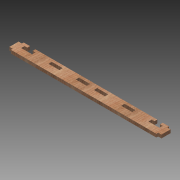
# Autodesk Inventor part: Viga trasera
Saved by Autodesk Inventor 2015 (Build 190159000, 159)
## iProperties
Created: 2016-02-08
Part Number: Viga trasera
Material: Wood (Birch)
Document SubType Name: Modeling
Designer: iberopuebla
Density: 0.55 g/cm^3
Appearance: Birch - Natural Polished
Author: iberopuebla
Autodesk Inventor part; units mm, degrees
ref_plane "YZ Plane" through (0, 0, 0) normal (1, 0, 0) x (0, 1, 0)
ref_plane "XZ Plane" through (0, 0, 0) normal (0, 1, 0) x (-1, 0, 0)
ref_plane "XY Plane" through (0, 0, 0) normal (0, 0, 1) x (1, 0, 0)
sketch "Sketch1" plane through (0, 0, 0) normal (0, 0, 1) x (1, 0, 0)
  line L0 (-2761.2962, 915.5779) -> (-1961.2962, 915.5779)
  line L1 (-1961.2962, 845.5779) -> (-2761.2962, 845.5779)
  line L2 (-2761.2962, 905.5779) -> (-2779.2962, 905.5779)
  line L3 (-2779.2962, 905.5779) -> (-2779.2962, 855.5779)
  line L4 (-2779.2962, 855.5779) -> (-2761.2962, 855.5779)
  line L5 (-1961.2962, 905.5779) -> (-1943.2962, 905.5779)
  line L6 (-1943.2962, 905.5779) -> (-1943.2962, 855.5779)
  line L7 (-1943.2962, 855.5779) -> (-1961.2962, 855.5779)
  line L8 (-1961.2962, 915.5779) -> (-1961.2962, 905.5779)
  line L9 (-1961.2962, 855.5779) -> (-1961.2962, 845.5779)
  line L10 (-2761.2962, 845.5779) -> (-2761.2962, 855.5779)
  line L11 (-2761.2962, 905.5779) -> (-2761.2962, 915.5779)
  point P0 (0, 0)
  dimension "d8" = 800
  dimension "d9" = 70
  dimension "d11" = 50
  dimension "d12" = 18
  dimension "d13" = 18
  dimension "d14" = 50
  dimension "d15" = 10
  dimension "d18" = 800
  dimension "d19" = 10
  dimension "d20" = 10
  constraints: 24 end point, 7 parallel, 4 perpendicular, 3 horizontal
  measures "d8" distance of L0.start L0.end
  measures "d9" distance between parallel lines of L1 L0
  measures "d11" distance of L2.start L4.end
  measures "d12" distance of L3.end L4.end
  measures "d13" distance of L5.start L5.end
  measures "d14" distance of L5.end L6.end
  measures "d15" distance between parallel lines of L0 L5
  measures "d18" distance of L1.start L1.end
  measures "d19" distance between parallel lines of L0 L2
  measures "d20" distance between parallel lines of L1 L4
extrude "Extrusion1" add sketch "Sketch1" along normal blind 18
sketch "Sketch2" plane through (0, 0, 18) normal (0, 0, 1) x (1, 0, 0)
  line L0 (-1961.2962, 905.5779) -> (-1960.1648, 906.7093)
  line L1 (-1961.2962, 905.5779) -> (-1959.6962, 905.5779) construction
  line L2 (-1961.2962, 855.5779) -> (-1960.1648, 854.4466)
  line L3 (-2761.2962, 855.5779) -> (-2762.4276, 854.4466)
  line L4 (-2761.2962, 905.5779) -> (-2762.4276, 906.7093)
  circle A0 centre (-2762.4276, 906.7093) radius 1.6
  circle A1 centre (-2762.4276, 854.4466) radius 1.6
  circle A2 centre (-1960.1648, 906.7093) radius 1.6
  circle A3 centre (-1960.1648, 854.4466) radius 1.6
  line L5 (-1943.2962, 855.5779) -> (-1943.2962, 905.5779) projected
  line L6 (-2779.2962, 905.5779) -> (-2779.2962, 855.5779) projected
  point P0 (0, 0)
  dimension "d21" = 1.6
  dimension "d22" = 45
  dimension "d23" = 3.2
  dimension "d24" = 3.2
  dimension "d25" = 3.2
  dimension "d26" = 3.2
  dimension "d29" = 836
  constraints: 10 end point, 4 centre point, 3 coincident, 3 perpendicular, 1 equal length, 1 horizontal, 1 point on line
  measures "d21" distance of L0.start L0.end
  measures "d22" angle of L1 L0
  measures "d23" diameter of A0
  measures "d24" diameter of A1
  measures "d25" diameter of A2
  measures "d26" diameter of A3
  measures "d29" distance between parallel lines of L5 L6
extrude "Extrusion2" cut sketch "Sketch2" against normal blind 20
sketch "Sketch3" plane through (0, 0, 18) normal (0, 0, 1) x (1, 0, 0)
  line L0 (-2761.2962, 900.5779) -> (-1961.2962, 900.5779)
  line L1 (-1961.2962, 900.5779) -> (-1961.2962, 882.5779)
  line L2 (-1961.2962, 882.5779) -> (-2761.2962, 882.5779)
  line L3 (-2761.2962, 882.5779) -> (-2761.2962, 900.5779)
  line L4 (-2661.2962, 900.5779) -> (-2661.2962, 882.5779)
  line L5 (-2741.2962, 900.5779) -> (-2741.2962, 882.5779)
  line L6 (-2681.2962, 900.5779) -> (-2681.2962, 882.5779)
  line L7 (-2041.2962, 900.5779) -> (-2041.2962, 882.5779)
  line L8 (-1981.2962, 900.5779) -> (-1981.2962, 882.5779)
  line L9 (-2061.2962, 900.5779) -> (-2061.2962, 882.5779)
  line L10 (-2611.2962, 882.5779) -> (-2611.2962, 900.5779)
  line L11 (-2591.2962, 900.5779) -> (-2591.2962, 882.5779)
  line L12 (-2531.2962, 900.5779) -> (-2531.2962, 882.5779)
  line L13 (-2111.2962, 900.5779) -> (-2111.2962, 882.5779)
  line L14 (-2511.2962, 900.5779) -> (-2511.2962, 882.5779)
  line L15 (-2461.2962, 900.5779) -> (-2461.2962, 882.5779)
  line L16 (-2211.2962, 900.5779) -> (-2211.2962, 882.5779)
  line L17 (-2191.2962, 900.5779) -> (-2191.2962, 882.5779)
  line L18 (-2131.2962, 900.5779) -> (-2131.2962, 882.5779)
  line L19 (-2261.2962, 900.5779) -> (-2261.2962, 882.5779)
  line L20 (-2361.2962, 900.5779) -> (-2361.2962, 882.5779)
  line L21 (-2441.2962, 900.5779) -> (-2441.2962, 882.5779)
  line L22 (-2381.2962, 900.5779) -> (-2381.2962, 882.5779)
  line L23 (-2341.2962, 900.5779) -> (-2341.2962, 882.5779)
  line L24 (-2281.2962, 900.5779) -> (-2281.2962, 882.5779)
  line L25 (-1961.2962, 915.5779) -> (-2761.2962, 915.5779) projected
  line L26 (-2761.2962, 915.5779) -> (-2761.2962, 907.8407) projected
  point P0 (0, 0)
  dimension "d54" = 800
  dimension "d55" = 18
  dimension "d56" = 100
  dimension "d57" = 20
  dimension "d58" = 60
  dimension "d59" = 100
  dimension "d60" = 60
  dimension "d61" = 20
  dimension "d62" = 600
  dimension "d63" = 50
  dimension "d64" = 50
  dimension "d65" = 100
  dimension "d66" = 60
  dimension "d67" = 20
  dimension "d68" = 50
  dimension "d69" = 100
  dimension "d70" = 60
  dimension "d71" = 20
  dimension "d72" = 50
  dimension "d73" = 100
  dimension "d74" = 60
  dimension "d75" = 20
  dimension "d76" = 60
  dimension "d77" = 20
  dimension "d78" = 15
  dimension "d79" = 0
  constraints: 46 end point, 22 vertical, 1 parallel, 48 other
  measures "d54" distance of L1.end L3.start
  measures "d55" distance of L1.start L1.end
  measures "d56" distance between parallel lines of L3 L4
  measures "d57" distance between parallel lines of L3 L5
  measures "d58" distance between parallel lines of L6 L5
  measures "d59" distance between parallel lines of L9 L1
  measures "d60" distance between parallel lines of L8 L7
  measures "d61" distance between parallel lines of L9 L7
  measures "d62" distance between parallel lines of L9 L4
  measures "d63" distance between parallel lines of L10 L4
  measures "d64" distance between parallel lines of L13 L9
  measures "d65" distance between parallel lines of L10 L14
  measures "d66" distance from line of L12 L11.start
  measures "d67" distance between parallel lines of L10 L11
  measures "d68" distance between parallel lines of L14 L15
  measures "d69" distance between parallel lines of L13 L16
  measures "d70" distance between parallel lines of L18 L17
  measures "d71" distance between parallel lines of L16 L17
  measures "d72" distance between parallel lines of L16 L19
  measures "d73" distance between parallel lines of L15 L20
  measures "d74" distance between parallel lines of L21 L22
  measures "d75" distance between parallel lines of L15 L21
  measures "d76" distance between parallel lines of L24 L23
  measures "d77" distance between parallel lines of L23 L20
  measures "d79" distance between parallel lines of L3 L26
extrude "Extrusion3" cut sketch "Sketch3" against normal blind 20 contours L0 L6 L2 L5 | L0 L12 L2 L11 | L0 L22 L2 L21 | L0 L24 L2 L23 | L0 L18 L2 L17 | L0 L8 L2 L7
sketch "Sketch4" plane through (0, 0, 18) normal (0, 0, 1) x (1, 0, 0)
  line L0 (-2741.2962, 900.5779) -> (-2740.1648, 899.4466)
  line L1 (-2741.2962, 900.5779) -> (-2739.6962, 900.5779) construction
  line L2 (-2741.2962, 882.5779) -> (-2740.1648, 883.7093)
  line L3 (-2681.2962, 882.5779) -> (-2682.4276, 883.7093)
  line L4 (-2681.2962, 900.5779) -> (-2682.4276, 899.4466)
  line L5 (-2591.2962, 900.5779) -> (-2590.1648, 899.4466)
  line L6 (-2591.2962, 882.5779) -> (-2590.1648, 883.7093)
  line L7 (-2531.2962, 900.5779) -> (-2532.4276, 899.4466)
  line L8 (-2531.2962, 882.5779) -> (-2532.4276, 883.7093)
  line L9 (-2441.2962, 882.5779) -> (-2440.1648, 883.7093)
  line L10 (-2441.2962, 882.5779) -> (-2439.6962, 882.5779) construction
  line L11 (-2441.2962, 900.5779) -> (-2440.1648, 899.4466)
  line L12 (-2381.2962, 900.5779) -> (-2382.4276, 899.4466)
  line L13 (-2381.2962, 882.5779) -> (-2382.4276, 883.7093)
  line L14 (-2341.2962, 900.5779) -> (-2340.1648, 899.4466)
  line L15 (-2341.2962, 882.5779) -> (-2340.1648, 883.7093)
  line L16 (-2281.2962, 900.5779) -> (-2282.4276, 899.4466)
  line L17 (-2281.2962, 882.5779) -> (-2282.4276, 883.7093)
  line L18 (-2191.2962, 900.5779) -> (-2190.1648, 899.4466)
  line L19 (-2191.2962, 882.5779) -> (-2190.1648, 883.7093)
  line L20 (-2131.2962, 900.5779) -> (-2132.4276, 899.4466)
  line L21 (-2131.2962, 882.5779) -> (-2132.4276, 883.7093)
  line L22 (-2041.2962, 900.5779) -> (-2040.1648, 899.4466)
  line L23 (-2041.2962, 882.5779) -> (-2040.1648, 883.7093)
  line L24 (-1981.2962, 900.5779) -> (-1982.4276, 899.4466)
  line L25 (-1981.2962, 882.5779) -> (-1982.4276, 883.7093)
  circle A0 centre (-2040.1648, 899.4466) radius 1.6
  circle A1 centre (-2040.1648, 883.7093) radius 1.6
  circle A2 centre (-1982.4276, 899.4466) radius 1.6
  circle A3 centre (-1982.4276, 883.7093) radius 1.6
  circle A4 centre (-2132.4276, 899.4466) radius 1.6
  circle A5 centre (-2132.4276, 883.7093) radius 1.6
  circle A6 centre (-2190.1648, 899.4466) radius 1.6
  circle A7 centre (-2190.1648, 883.7093) radius 1.6
  circle A8 centre (-2282.4276, 899.4466) radius 1.6
  circle A9 centre (-2282.4276, 883.7093) radius 1.6
  circle A10 centre (-2340.1648, 899.4466) radius 1.6
  circle A11 centre (-2340.1648, 883.7093) radius 1.6
  circle A12 centre (-2382.4276, 899.4466) radius 1.6
  circle A13 centre (-2382.4276, 883.7093) radius 1.6
  circle A14 centre (-2440.1648, 899.4466) radius 1.6
  circle A15 centre (-2440.1648, 883.7093) radius 1.6
  circle A16 centre (-2532.4276, 899.4466) radius 1.6
  circle A17 centre (-2532.4276, 883.7093) radius 1.6
  circle A18 centre (-2590.1648, 899.4466) radius 1.6
  circle A19 centre (-2590.1648, 883.7093) radius 1.6
  circle A20 centre (-2682.4276, 899.4466) radius 1.6
  circle A21 centre (-2682.4276, 883.7093) radius 1.6
  circle A22 centre (-2740.1648, 899.4466) radius 1.6
  circle A23 centre (-2740.1648, 883.7093) radius 1.6
  point P0 (0, 0)
  dimension "d62" = 600
  dimension "d82" = 1.6
  dimension "d83" = 45
  dimension "d84" = 1.6
  dimension "d85" = 45
  dimension "d86" = 3.2
  dimension "d87" = 3.2
  dimension "d88" = 3.2
  dimension "d89" = 3.2
  dimension "d90" = 3.2
  dimension "d91" = 3.2
  dimension "d92" = 3.2
  dimension "d93" = 3.2
  dimension "d94" = 3.2
  dimension "d95" = 3.2
  dimension "d96" = 3.2
  dimension "d97" = 3.2
  dimension "d98" = 3.2
  dimension "d99" = 3.2
  dimension "d100" = 3.2
  dimension "d101" = 3.2
  dimension "d102" = 3.2
  dimension "d103" = 3.2
  dimension "d104" = 3.2
  dimension "d105" = 3.2
  dimension "d106" = 3.2
  dimension "d107" = 3.2
  dimension "d108" = 3.2
  dimension "d109" = 3.2
  constraints: 52 end point, 46 coincident, 24 centre point, 15 perpendicular, 7 parallel, 2 equal length, 2 horizontal, 2 point on line
  measures "d82" distance of L0.start L0.end
  measures "d83" angle of L0 L1
  measures "d84" distance of L9.start L9.end
  measures "d85" angle of L10 L9
  measures "d86" diameter of A0
  measures "d87" diameter of A1
  measures "d88" diameter of A2
  measures "d89" diameter of A3
  measures "d90" diameter of A4
  measures "d91" diameter of A5
  measures "d92" diameter of A6
  measures "d93" diameter of A7
  measures "d94" diameter of A8
  measures "d95" diameter of A9
  measures "d96" diameter of A10
  measures "d97" diameter of A11
  measures "d98" diameter of A12
  measures "d99" diameter of A13
  measures "d100" diameter of A14
  measures "d101" diameter of A15
  measures "d102" diameter of A16
  measures "d103" diameter of A17
  measures "d104" diameter of A18
  measures "d105" diameter of A19
  measures "d106" diameter of A20
  measures "d107" diameter of A21
  measures "d108" diameter of A22
  measures "d109" diameter of A23
extrude "Extrusion4" cut sketch "Sketch4" against normal blind 20
sketch "Sketch5" plane through (0, 0, 18) normal (0, 0, 1) x (1, 0, 0)
  line L0 (-2761.2962, 915.5779) -> (-1961.2962, 915.5779) projected
  line L1 (-2683.559, 900.5779) -> (-2739.0335, 900.5779) projected
  line L2 (-2726.2962, 915.5779) -> (-2696.2962, 915.5779)
  line L3 (-2696.2962, 915.5779) -> (-2696.2962, 900.5779)
  line L4 (-2696.2962, 900.5779) -> (-2726.2962, 900.5779)
  line L5 (-2726.2962, 900.5779) -> (-2726.2962, 915.5779)
  line L6 (-2761.2962, 915.5779) -> (-2761.2962, 907.8407) projected
  line L7 (-2741.2962, 884.8407) -> (-2741.2962, 898.3152) projected
  line L8 (-1961.2962, 915.5779) -> (-2761.2962, 915.5779) projected
  line L9 (-2039.0335, 900.5779) -> (-1983.559, 900.5779) projected
  line L10 (-1996.2962, 915.5779) -> (-2026.2962, 915.5779)
  line L11 (-2026.2962, 915.5779) -> (-2026.2962, 900.5779)
  line L12 (-2026.2962, 900.5779) -> (-1996.2962, 900.5779)
  line L13 (-1996.2962, 900.5779) -> (-1996.2962, 915.5779)
  line L14 (-1981.2962, 898.3152) -> (-1981.2962, 884.8407) projected
  point P0 (0, 0)
  dimension "d112" = 30
  dimension "d114" = 15
  dimension "d115" = 30
  dimension "d116" = 15
  constraints: 16 end point, 4 parallel, 4 point on line, 2 horizontal, 2 perpendicular
  measures "d112" distance of L3.end L4.end
  measures "d114" distance between parallel lines of L5 L7
  measures "d115" distance of L12.end L11.end
  measures "d116" distance between parallel lines of L13 L14
extrude "Extrusion5" cut sketch "Sketch5" against normal blind 20
body "Solid1"
